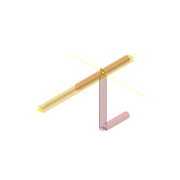
# Autodesk Inventor part: cellSTORM_laserbeam
Saved by Autodesk Inventor 2019.4 (Build 234330000, 330)
## iProperties
Created: 2020-04-17
Part Number: cellSTORM_laserbeam
Material: Generic
Document SubType Name: Modeling
Designer: diederichbenedict
Density: 1 g/cm^3
Appearance: Polycarbonate - Clear
Author: diederichbenedict
Autodesk Inventor part; units mm, degrees
ref_plane "YZ Plane" through (0, 0, 0) normal (1, 0, 0) x (0, 1, 0)
ref_plane "XY Plane" through (0, 0, 0) normal (0, 0, 1) x (1, 0, 0)
sketch "Sketch1" plane through (0, 0, 0) normal (0, 0, 1) x (1, 0, 0)
  circle A0 centre (0, 0) radius 6 projected
  circle A1 centre (0, 0) radius 2
  point P0 (0, 0)
  dimension "d0" = 4
  constraints: 1 centre point
  measures "d0" radial gap between concentric circles of A0 A1
ref_plane "Work Plane1" through (-3.5125, -3.5125, 37.5) normal (0, 0, 1) x (0.9086751, 0.417504, 0)
extrude "Extrusion1" add sketch "Sketch1" along normal up to surface (37.5 mm away) contours A1
sketch "Sketch2" plane through (0, 0, 37.5) normal (0, 0, 1) x (1, 0, 0)
  circle A0 centre (0, 0) radius 2 projected
  point P0 (0, 0)
extrude "Extrusion2" add sketch "Sketch2" along normal blind 2 draft -40
sketch "Sketch3" plane through (0, 0, 39.5) normal (0, 0, 1) x (1, 0, 0)
  circle A0 centre (0, 0) radius 0.3218 projected
  point P0 (0, 0)
ref_plane "Work Plane2" through (-0.9, -20.4499, 62.8) normal (0, 0, 1) x (1, 0, 0)
extrude "Extrusion3" add sketch "Sketch3" along normal up to surface (23.3 mm away)
ref_plane "Work Plane3" through (0, 0, 18.5) normal (0, 0, -1) x (-1, 0, 0)
sketch "Sketch4" plane through (0, 0, 18.5) normal (0, 0, -1) x (-1, 0, 0)
  point P0 (0, 0)
ref_plane "Work Plane4" through (0, -2, 0) normal (0, 1, 0) x (-1, 0, 0)
sketch "Sketch5" plane through (0, -2, 0) normal (0, 1, 0) x (-1, 0, 0)
  line L0 (-2, 37.5) -> (2, 37.5) projected
  line L1 (-2, 0) -> (2, 0) projected
  line L2 (-2, 0) -> (-2, 37.5) projected
  line L3 (2, 0) -> (2, 37.5) projected
  circle A0 centre (0, 18.5) radius 2
  point P0 (0, 0)
  constraints: 1 centre point, 1 tangent
extrude "Extrusion4" add sketch "Sketch5" along normal blind 2 and the other way blind 35 contours A0
sketch "Sketch6" plane through (0, 0, 0) normal (0, 0, -1) x (-1, 0, 0)
  arc A0 (-2, 0) -> (2, 0) centre (0, 0) ccw projected
  arc A1 (-2, 0) -> (2, 0) centre (0, 0) ccw projected
  line L0 (-2, -37) -> (2, -37) projected
  line L1 (-2, -37) -> (2, -37) projected
  circle A2 centre (0, -37) radius 2
  point P0 (0, 0)
  constraints: 1 horizontal alignment, 1 midpoint, 2 other
extrude "Extrusion5" add sketch "Sketch6" against normal up to surface round surface about axis through (0, -2, 18.5) along (0, 1, 0) radius 2 far side no
ref_plane "Work Plane8" through (0, 0, 18.5) normal (0, 0.7071068, -0.7071068) x (1, 0, 0)
ref_plane "Work Plane7" through (0, 0, 66.1774) normal (0, 1, 0) x (-1, 0, 0)
ref_plane "Work Plane6" through (-4.3067, 1.9434, 62.8114) normal (0, 0.8660254, 0.5) x (1, 0, 0)
body "Solid1"
